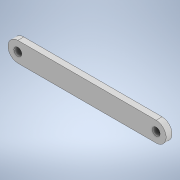
# Autodesk Inventor part: 零件3
Saved by Autodesk Inventor 2022 (Build 260153000, 153)
## iProperties
Created: 2023-04-16
Part Number: 零件3
Material: 一般
Document SubType Name: Modeling
Designer: JOU
Density: 1 g/cm^3
Appearance: 預設
Author: JOU
Autodesk Inventor part; units mm, degrees
ref_plane "YZ Plane" through (0, 0, 0) normal (1, 0, 0) x (0, 1, 0)
ref_plane "XZ Plane" through (0, 0, 0) normal (0, 1, 0) x (-1, 0, 0)
ref_plane "XY Plane" through (0, 0, 0) normal (0, 0, 1) x (1, 0, 0)
sketch "草圖1" plane through (0, 0, 0) normal (0, 0, 1) x (1, 0, 0)
  line L0 (0, 0) -> (-70, 0) construction
  line L1 (0, 5) -> (-70, 5)
  line L2 (-70, -5) -> (0, -5)
  arc A0 (0, -5) -> (0, 5) centre (0, 0) ccw
  arc A1 (-70, 5) -> (-70, -5) centre (-70, 0) ccw
  circle A2 centre (-70, 0) radius 2
  circle A3 centre (0, 0) radius 2
  point P0 (-35, 0)
  dimension "d0" = 70
  dimension "d1" = 4
  dimension "d2" = 4
  dimension "d3" = 10
  constraints: 8 end point, 4 centre point, 4 point on circle, 4 tangent, 2 coincident, 1 horizontal, 1 midpoint, 1 parallel
  measures "d0" distance of L1.start L1.end
  measures "d1" diameter of A2
  measures "d2" diameter of A3
  measures "d3" distance between parallel lines of L2 L1
extrude "擠出1" add sketch "草圖1" along normal blind 3
